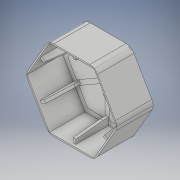
# Autodesk Inventor part: Base v5 - 175
Saved by Autodesk Inventor 2019 (Build 230136000, 136)
## iProperties
Created: 2021-07-14
Part Number: Base v5 - 175
Material: Generic
Document SubType Name: Modeling
Designer: Lix
Density: 1 g/cm^3
Appearance: Default
Author: Lix
## iProperties of the stored document Base v6 - 175_3DPrint.ipt
Created: 2021-08-07
Part Number: Base v6 - 175_3DPrint
Material: Generic
Document SubType Name: Modeling
Designer: Lix
Density: 1 g/cm^3
Appearance: Default
Author: Lix
Autodesk Inventor part; units mm, degrees
sketch "Sketch1" plane through (0, 0, 0) normal (0, 0, 1) x (1, 0, 0)
  line L0 (25.4034, -44) -> (-25.4034, -44)
  line L1 (-25.4034, -44) -> (-50.8068, 0)
  line L2 (-50.8068, 0) -> (-25.4034, 44)
  line L3 (-25.4034, 44) -> (25.4034, 44)
  line L4 (25.4034, 44) -> (50.8068, 0)
  line L5 (50.8068, 0) -> (25.4034, -44)
  point P0 (0, 0)
  point P1 (0, 0)
  point P2 (0, 0)
  dimension "d0" = 88
  constraints: 12 end point, 2 coincident, 1 horizontal, 13 other
  measures "d0" distance between parallel lines of L5 L2
extrude "Extrusion1" add sketch "Sketch1" along normal blind 40
shell "Shell1" thickness 1.5 removed faces 1 at (-8.4678, 14.6667, 40) ; own thickness 1 on faces at (-8.4678, 14.6667, 0)
sketch "Sketch11" plane through (-24.5374, -42.5, 1) normal (0, 0, 1) x (1, 0, 0)
  line L0 (-41.7126, -1) -> (-30.7126, -1)
  line L1 (-30.7126, -1) -> (-30.7126, 86)
  line L2 (-30.7126, 86) -> (-41.7126, 86)
  line L3 (-41.7126, 86) -> (-41.7126, -1)
  line L4 (-41.7126, -1) -> (-30.7126, 86) construction
  line L5 (-30.7126, -1) -> (-41.7126, 86) construction
  line L6 (-1.2126, -1) -> (9.7874, -1)
  line L7 (9.7874, -1) -> (9.7874, 86)
  line L8 (9.7874, 86) -> (-1.2126, 86)
  line L9 (-1.2126, -1) -> (9.7874, 86) construction
  line L10 (9.7874, -1) -> (-1.2126, 86) construction
  line L11 (-1.2126, 86) -> (-1.2126, -1)
  line L12 (39.2874, -1) -> (50.2874, -1)
  line L13 (50.2874, -1) -> (50.2874, 86)
  line L14 (50.2874, 86) -> (39.2874, 86)
  line L15 (39.2874, -1) -> (50.2874, 86) construction
  line L16 (50.2874, -1) -> (39.2874, 86) construction
  line L17 (39.2874, 86) -> (39.2874, -1)
  line L18 (79.7874, -1) -> (90.7874, -1)
  line L19 (90.7874, -1) -> (90.7874, 86)
  line L20 (90.7874, 86) -> (79.7874, 86)
  line L21 (79.7874, -1) -> (90.7874, 86) construction
  line L22 (90.7874, -1) -> (79.7874, 86) construction
  line L23 (79.7874, 86) -> (79.7874, -1)
  line L24 (-36.2126, 42.5) -> (85.2874, 42.5) construction
  line L25 (-18.9626, -28) -> (68.0374, -28)
  line L26 (68.0374, -28) -> (68.0374, -17)
  line L27 (68.0374, -17) -> (-18.9626, -17)
  line L28 (-18.9626, -17) -> (-18.9626, -28)
  line L29 (-18.9626, -28) -> (68.0374, -17) construction
  line L30 (68.0374, -28) -> (-18.9626, -17) construction
  line L31 (24.5374, -22.5) -> (24.5374, 107.5) construction
  line L32 (-18.9626, 102) -> (68.0374, 102)
  line L33 (68.0374, 102) -> (68.0374, 113)
  line L34 (68.0374, 113) -> (-18.9626, 113)
  line L35 (-18.9626, 113) -> (-18.9626, 102)
  line L36 (-18.9626, 102) -> (68.0374, 113) construction
  line L37 (68.0374, 102) -> (-18.9626, 113) construction
  line L38 (-19.9626, 114) -> (69.0374, 114)
  line L39 (69.0374, 114) -> (69.0374, 101)
  line L40 (69.0374, 101) -> (-19.9626, 101)
  line L41 (-19.9626, 101) -> (-19.9626, 114)
  line L42 (-42.7126, 87) -> (-29.7126, 87)
  line L43 (-29.7126, 87) -> (-29.7126, -2)
  line L44 (-29.7126, -2) -> (-42.7126, -2)
  line L45 (-42.7126, -2) -> (-42.7126, 87)
  line L46 (-2.2126, 87) -> (10.7874, 87)
  line L47 (10.7874, 87) -> (10.7874, -2)
  line L48 (10.7874, -2) -> (-2.2126, -2)
  line L49 (-2.2126, -2) -> (-2.2126, 87)
  line L50 (38.2874, 87) -> (51.2874, 87)
  line L51 (51.2874, 87) -> (51.2874, -2)
  line L52 (51.2874, -2) -> (38.2874, -2)
  line L53 (38.2874, -2) -> (38.2874, 87)
  line L54 (78.7874, 87) -> (91.7874, 87)
  line L55 (91.7874, 87) -> (91.7874, -2)
  line L56 (91.7874, -2) -> (78.7874, -2)
  line L57 (78.7874, -2) -> (78.7874, 87)
  line L58 (69.0374, -29) -> (-19.9626, -29)
  line L59 (-19.9626, -29) -> (-19.9626, -16)
  line L60 (-19.9626, -16) -> (69.0374, -16)
  line L61 (69.0374, -16) -> (69.0374, -29)
  line L62 (90.7874, 87) -> (79.7874, 87)
  line L63 (79.7874, 87) -> (79.7874, -2)
  line L64 (79.7874, -2) -> (90.7874, -2)
  line L65 (90.7874, -2) -> (90.7874, 87)
  line L66 (50.2874, 87) -> (39.2874, 87)
  line L67 (39.2874, 87) -> (39.2874, -2)
  line L68 (39.2874, -2) -> (50.2874, -2)
  line L69 (50.2874, -2) -> (50.2874, 87)
  line L70 (69.0374, 113) -> (-19.9626, 113)
  line L71 (-19.9626, 113) -> (-19.9626, 102)
  line L72 (-19.9626, 102) -> (69.0374, 102)
  line L73 (69.0374, 102) -> (69.0374, 113)
  line L74 (-30.7126, 87) -> (-41.7126, 87)
  line L75 (-41.7126, 87) -> (-41.7126, -2)
  line L76 (-41.7126, -2) -> (-30.7126, -2)
  line L77 (-30.7126, -2) -> (-30.7126, 87)
  line L78 (9.7874, 87) -> (-1.2126, 87)
  line L79 (-1.2126, 87) -> (-1.2126, -2)
  line L80 (-1.2126, -2) -> (9.7874, -2)
  line L81 (9.7874, -2) -> (9.7874, 87)
  line L82 (69.0374, -17) -> (-19.9626, -17)
  line L83 (-19.9626, -17) -> (-19.9626, -28)
  line L84 (-19.9626, -28) -> (69.0374, -28)
  line L85 (69.0374, -28) -> (69.0374, -17)
  point P0 (24.5374, 42.5)
  point P1 (4.2874, 42.5)
  point P2 (44.7874, 42.5)
  point P3 (24.5374, 42.5)
  dimension "d138" = 11
  dimension "d139" = 87
  dimension "d142" = 40.5
  dimension "d147" = 130
  dimension "d151" = 1
  dimension "d152" = 1
  dimension "d153" = 1
  dimension "d154" = 1
  dimension "d155" = 1
  dimension "d156" = 1
  constraints: 172 end point, 24 parallel, 14 midpoint, 13 point on line, 12 perpendicular, 11 horizontal, 4 equal length, 1 coincident, 1 collinear, 1 horizontal alignment, 1 vertical, 50 other
  measures "d138" distance of L1.end L2.end
  measures "d139" distance of L2.end L0.start
  measures "d142" distance of L0.end L6.end
  measures "d147" distance of L31.start L31.end
  measures "d151" distance between parallel lines of L34 L38
  measures "d152" distance between parallel lines of L2 L42
  measures "d153" distance between parallel lines of L8 L46
  measures "d154" distance between parallel lines of L14 L50
  measures "d155" distance between parallel lines of L20 L54
  measures "d156" distance between parallel lines of L25 L58
extrude "Extrusion9" [suppressed]
ref_plane "Work Plane1" through (-12.7017, 22, 40) normal (0.8660254, 0.5, 0) x (0, 0, -1)
ref_plane "Work Plane2" through (-25.4034, 0, 0) normal (0, 1, 0) x (1, 0, 0)
ref_plane "Work Plane3" through (-12.7017, -22, 0) normal (-0.8660254, 0.5, 0) x (0, 0, 1)
sketch "Sketch12" plane through (-24.5374, -42.5, 1) normal (0, 0, 1) x (1, 0, 0)
  line L0 (49.0748, 0) -> (0, 0) projected
  line L1 (73.6122, 42.5) -> (49.0748, 0) projected
  line L2 (49.0748, 85) -> (73.6122, 42.5) projected
  line L3 (0, 85) -> (49.0748, 85) projected
  line L4 (-24.5374, 42.5) -> (0, 85) projected
  line L5 (0, 0) -> (-24.5374, 42.5) projected
  point P0 (24.5374, 42.5)
sketch "Sketch4" plane through (-24.5374, -42.5, 1) normal (0, 0, 1) x (1, 0, 0)
  line L0 (49.0748, 0) -> (0, 0) projected
  line L1 (73.6122, 42.5) -> (49.0748, 0) projected
  line L2 (49.0748, 85) -> (73.6122, 42.5) projected
  line L3 (0, 85) -> (49.0748, 85) projected
  line L4 (-24.5374, 42.5) -> (0, 85) projected
  line L5 (0, 0) -> (-24.5374, 42.5) projected
  line L6 (-6.7257, 63.3507) -> (2.8868, 80)
  line L7 (2.8868, 80) -> (22.1117, 80)
  line L8 (49.0748, 85) -> (0, 0) construction
  arc A0 (22.1117, 52.2014) -> (17.3486, 49.4514) centre (24.5374, 42.5) ccw
  line L9 (-6.7257, 63.3507) -> (17.3486, 49.4514)
  line L10 (22.1117, 80) -> (22.1117, 52.2014)
  circle A1 centre (49.6521, 86) radius 2.5
  arc A2 (14.9229, 45.25) -> (14.9229, 39.75) centre (24.5374, 42.5) ccw
  line L11 (-9.1514, 59.1493) -> (14.9229, 45.25)
  line L12 (-9.1514, 25.8507) -> (14.9229, 39.75)
  line L13 (-9.1514, 25.8507) -> (-18.7639, 42.5)
  line L14 (-18.7639, 42.5) -> (-9.1514, 59.1493)
  arc A3 (17.3486, 35.5486) -> (22.1117, 32.7986) centre (24.5374, 42.5) ccw
  line L15 (-6.7257, 21.6493) -> (17.3486, 35.5486)
  line L16 (22.1117, 5) -> (22.1117, 32.7986)
  line L17 (22.1117, 5) -> (2.8868, 5)
  line L18 (2.8868, 5) -> (-6.7257, 21.6493)
  arc A4 (26.963, 32.7986) -> (31.7262, 35.5486) centre (24.5374, 42.5) ccw
  line L19 (26.963, 5) -> (26.963, 32.7986)
  line L20 (55.8005, 21.6493) -> (31.7262, 35.5486)
  line L21 (55.8005, 21.6493) -> (46.188, 5)
  line L22 (46.188, 5) -> (26.963, 5)
  arc A5 (34.1518, 39.75) -> (34.1518, 45.25) centre (24.5374, 42.5) ccw
  line L23 (58.2262, 25.8507) -> (34.1518, 39.75)
  line L24 (58.2262, 59.1493) -> (34.1518, 45.25)
  line L25 (58.2262, 59.1493) -> (67.8387, 42.5)
  line L26 (67.8387, 42.5) -> (58.2262, 25.8507)
  arc A6 (31.7262, 49.4514) -> (26.963, 52.2014) centre (24.5374, 42.5) ccw
  line L27 (55.8005, 63.3507) -> (31.7262, 49.4514)
  line L28 (26.963, 80) -> (26.963, 52.2014)
  line L29 (26.963, 80) -> (46.188, 80)
  line L30 (46.188, 80) -> (55.8005, 63.3507)
  point P0 (-24.5374, 42.5)
  point P1 (0, 0)
  point P2 (49.0748, 0)
  point P3 (73.6122, 42.5)
  point P4 (49.0748, 85)
  dimension "d37" = 5
  dimension "d44" = 10
  dimension "d45" = 60
  dimension "d46" = 90
  dimension "d47" = 90
  dimension "d52" = 5.5
  dimension "d55" = 5
  dimension "d72" = 360
  constraints: 50 end point, 12 point on circle, 7 centre point, 2 equal length, 1 coincident, 1 midpoint, 73 other
  measures "d37" distance between parallel lines of L3 L7
  measures "d44" radius of A0
  measures "d45" angle of L10 L9
  measures "d46" angle of L9 L6
  measures "d47" angle of L10 L7
  measures "d52" distance of L10.end L9.end
  measures "d55" diameter of A1
extrude "Extrusion5" cut sketch "Sketch4" against normal blind 0.01 contours A1 L3 L2 | L2 L3 A1 | L6 L7 L10 A0 L9 | A2 L12 L13 L14 L11 | A3 L16 L17 L18 L15 | A4 L20 L21 L22 L19 | A5 L24 L25 L26 L23 | A6 L28 L29 L30 L27
sketch "Sketch8" plane through (-24.5374, -42.5, 1) normal (0, 0, 1) x (1, 0, 0)
  line L0 (49.0748, 0) -> (0, 0) projected
  line L1 (73.6122, 42.5) -> (49.0748, 0) projected
  line L2 (-24.5374, 42.5) -> (0, 85) projected
  line L3 (0, 0) -> (-24.5374, 42.5) projected
  line L4 (23.0374, 77) -> (26.0374, 77)
  line L5 (26.0374, 77) -> (26.0374, 85)
  line L6 (26.0374, 85) -> (23.0374, 85)
  line L7 (23.0374, 85) -> (23.0374, 77)
  line L8 (0, 85) -> (49.0748, 85) projected
  line L9 (24.5374, 86) -> (24.5374, 85)
  line L10 (58.2262, 25.8507) -> (34.1518, 39.75) projected
  arc A0 (34.1518, 39.75) -> (34.1518, 45.25) centre (24.5374, 42.5) ccw projected
  line L11 (34.1518, 45.25) -> (58.2262, 59.1493) projected
  line L12 (55.8005, 63.3507) -> (31.7262, 49.4514) projected
  arc A1 (31.7262, 49.4514) -> (26.963, 52.2014) centre (24.5374, 42.5) ccw projected
  line L13 (26.963, 52.2014) -> (26.963, 80) projected
  line L14 (26.963, 80) -> (46.188, 80) projected
  line L15 (2.8868, 80) -> (22.1117, 80) projected
  line L16 (22.1117, 80) -> (22.1117, 52.2014) projected
  arc A2 (22.1117, 52.2014) -> (17.3486, 49.4514) centre (24.5374, 42.5) ccw projected
  line L17 (17.3486, 49.4514) -> (-6.7257, 63.3507) projected
  line L18 (-9.1514, 59.1493) -> (14.9229, 45.25) projected
  arc A3 (14.9229, 45.25) -> (14.9229, 39.75) centre (24.5374, 42.5) ccw projected
  line L19 (14.9229, 39.75) -> (-9.1514, 25.8507) projected
  line L20 (-6.7257, 21.6493) -> (17.3486, 35.5486) projected
  arc A4 (17.3486, 35.5486) -> (22.1117, 32.7986) centre (24.5374, 42.5) ccw projected
  line L21 (22.1117, 32.7986) -> (22.1117, 5) projected
  line L22 (22.1117, 5) -> (2.8868, 5) projected
  line L23 (46.188, 5) -> (26.963, 5) projected
  line L24 (26.963, 5) -> (26.963, 32.7986) projected
  arc A5 (26.963, 32.7986) -> (31.7262, 35.5486) centre (24.5374, 42.5) ccw projected
  line L25 (31.7262, 35.5486) -> (55.8005, 21.6493) projected
  arc A6 (47.3608, 85) -> (49.9317, 83.5157) centre (49.6521, 86) ccw projected
  line L26 (0, 85) -> (47.3608, 85) projected
  line L27 (46.188, 80) -> (55.8005, 63.3507) projected
  line L28 (49.9317, 83.5157) -> (73.6122, 42.5) projected
  line L29 (55.8005, 21.6493) -> (46.188, 5) projected
  line L30 (58.2262, 59.1493) -> (67.8387, 42.5) projected
  line L31 (67.8387, 42.5) -> (58.2262, 25.8507) projected
  line L32 (2.8868, 5) -> (-6.7257, 21.6493) projected
  line L33 (-6.7257, 63.3507) -> (2.8868, 80) projected
  line L34 (-9.1514, 25.8507) -> (-18.7639, 42.5) projected
  line L35 (-18.7639, 42.5) -> (-9.1514, 59.1493) projected
  point P0 (24.5374, 42.5)
  dimension "d57" = 3
  dimension "d58" = 8
  constraints: 10 end point, 2 midpoint, 2 parallel, 1 coincident, 1 horizontal, 1 perpendicular, 1 vertical
  measures "d57" distance of L4.start L4.end
  measures "d58" distance of L4.end L5.end
extrude "Extrusion6" add sketch "Sketch8" along normal blind 36 contours L6 L5 L4 L7
sketch "Sketch9" plane through (1.5, 34.5, 1) normal (1, 0, 0) x (0, 0, -1)
  line L0 (0, 0) -> (0, 8) projected
  line L1 (0, 0) -> (-36, 0) projected
  line L2 (-36, 8) -> (-36, 0) projected
  line L3 (0, 8) -> (-36, 8) projected
  line L4 (-36, 8) -> (-36, 0) projected
  line L5 (-36, 0) -> (-6, 0)
  line L6 (0, 0) -> (-36, 0) projected
  line L7 (-6, 0) -> (-36, 3)
  line L8 (-36, 3) -> (-36, 0)
  point P0 (1, -34.5)
  point P1 (-36, 8)
  dimension "d77" = 3
  dimension "d78" = 30
  constraints: 6 end point, 3 point on line, 1 collinear, 1 perpendicular
  measures "d77" distance of L7.end L5.start
  measures "d78" distance of L5.start L5.end
extrude "Extrusion8" cut sketch "Sketch9" against normal blind 20 contours L1 L2 L7
pattern_circular "Circular Pattern1" count 6 over 360 about axis through (0, 0, 1) along (0, 0, -1) of "Extrusion6", "Extrusion8"
fillet "Fillet1" [suppressed]
fillet "Fillet2" radius 10 7 edges at (50.8068, 0, 20) (25.4034, 44, 0.495) (25.4034, 44, 20.5) (-25.4034, 44, 20) (25.4034, -44, 20) (-50.8068, 0, 20) (-25.4034, -44, 20)
fillet "Fillet4" radius 2 5 edges at (-7.1888, 6.9514, 0.995) (-2.4257, 9.7014, 0.995) (-2.4257, 37.5, 0.995) (-21.6506, 37.5, 0.995) (-31.2631, 20.8507, 0.995)
sketch "Sketch5" plane through (-19.6299, 44, 0) normal (0, 1, 0) x (1, 0, 0)
  line L0 (0, 0) -> (39.2598, 0) projected
  line L1 (0, -40) -> (0, 0) projected
  point P0 (19.6299, 0)
  point P1 (19.6299, -20)
  point P2 (19.6299, 0)
  point P3 (0, -20)
  constraints: 2 midpoint, 1 horizontal alignment, 1 vertical alignment
sketch "Sketch6" plane through (28.2902, 39, 40) normal (0.8660254, 0.5, 0) x (0, 0, -1)
  line L0 (40, 8.6603) -> (0, 8.6603) projected
  point P0 (40, -19.6299)
  point P1 (20, -19.6299)
  point P2 (20, 8.6603)
  constraints: 1 horizontal alignment, 1 midpoint, 1 vertical alignment
sketch "Sketch7" plane through (28.2902, -39, 40) normal (0.8660254, -0.5, 0) x (0, 0, -1)
  line L0 (0, -8.6603) -> (40, -8.6603) projected
  point P0 (40, 19.6299)
  point P1 (20, 19.6299)
  point P2 (20, -8.6603)
  constraints: 1 horizontal alignment, 1 midpoint, 1 vertical alignment
sketch "Sketch13" plane through (0, 0, 40) normal (0, 0, 1) x (1, 0, 0)
  line L0 (-66.25, -43.5) -> (-55.25, -43.5) projected
  line L1 (-55.25, -43.5) -> (-55.25, 43.5) projected
  line L2 (-55.25, 43.5) -> (-66.25, 43.5) projected
  line L3 (-66.25, 43.5) -> (-66.25, -43.5) projected
  line L4 (-25.75, -43.5) -> (-14.75, -43.5) projected
  line L5 (-14.75, -43.5) -> (-14.75, 43.5) projected
  line L6 (-14.75, 43.5) -> (-25.75, 43.5) projected
  line L7 (-25.75, 43.5) -> (-25.75, -43.5) projected
  line L8 (-43.5, 59.5) -> (43.5, 59.5) projected
  line L9 (43.5, 59.5) -> (43.5, 70.5) projected
  line L10 (43.5, 70.5) -> (-43.5, 70.5) projected
  line L11 (-43.5, 70.5) -> (-43.5, 59.5) projected
  line L12 (14.75, -43.5) -> (25.75, -43.5) projected
  line L13 (25.75, -43.5) -> (25.75, 43.5) projected
  line L14 (25.75, 43.5) -> (14.75, 43.5) projected
  line L15 (14.75, 43.5) -> (14.75, -43.5) projected
  line L16 (55.25, -43.5) -> (66.25, -43.5) projected
  line L17 (66.25, -43.5) -> (66.25, 43.5) projected
  line L18 (66.25, 43.5) -> (55.25, 43.5) projected
  line L19 (55.25, 43.5) -> (55.25, -43.5) projected
  line L20 (-43.5, -70.5) -> (43.5, -70.5) projected
  line L21 (43.5, -70.5) -> (43.5, -59.5) projected
  line L22 (43.5, -59.5) -> (-43.5, -59.5) projected
  line L23 (-43.5, -59.5) -> (-43.5, -70.5) projected
  arc A0 (-28.2902, -39) -> (-19.6299, -44) centre (-19.6299, -34) ccw projected
  line L24 (-19.6299, -44) -> (19.6299, -44) projected
  arc A1 (19.6299, -44) -> (28.2902, -39) centre (19.6299, -34) ccw projected
  line L25 (28.2902, -39) -> (47.9201, -5) projected
  arc A2 (47.9201, -5) -> (47.9201, 5) centre (39.2598, 0) ccw projected
  line L26 (47.9201, 5) -> (28.2902, 39) projected
  arc A3 (28.2902, 39) -> (19.6299, 44) centre (19.6299, 34) ccw projected
  line L27 (19.6299, 44) -> (-19.6299, 44) projected
  arc A4 (-19.6299, 44) -> (-28.2902, 39) centre (-19.6299, 34) ccw projected
  line L28 (-28.2902, 39) -> (-47.9201, 5) projected
  arc A5 (-47.9201, 5) -> (-47.9201, -5) centre (-39.2598, 0) ccw projected
  line L29 (-47.9201, -5) -> (-28.2902, -39) projected
  line L30 (-24.5374, -42.5) -> (-49.0748, 0) projected
  line L31 (-49.0748, 0) -> (-24.5374, 42.5) projected
  line L32 (-24.5374, 42.5) -> (24.5374, 42.5) projected
  line L33 (24.5374, 42.5) -> (49.0748, 0) projected
  line L34 (49.0748, 0) -> (24.5374, -42.5) projected
  line L35 (24.5374, -42.5) -> (-24.5374, -42.5) projected
  line L36 (1.5, -37.5) -> (-1.5, -37.5) projected
  line L37 (-1.5, -37.5) -> (-1.5, -42.5) projected
  line L38 (1.5, -42.5) -> (-1.5, -42.5) projected
  line L39 (1.5, -42.5) -> (1.5, -37.5) projected
  line L40 (-31.726, -20.049) -> (-33.226, -17.451) projected
  line L41 (-33.226, -17.451) -> (-37.5561, -19.951) projected
  line L42 (-36.0561, -22.549) -> (-37.5561, -19.951) projected
  line L43 (-36.0561, -22.549) -> (-31.726, -20.049) projected
  line L44 (-29.1279, -18.549) -> (-31.726, -20.049) projected
  line L45 (-30.6279, -15.951) -> (-29.1279, -18.549) projected
  line L46 (-33.226, -17.451) -> (-30.6279, -15.951) projected
  line L47 (-31.726, -20.049) -> (-33.226, -17.451) projected
  line L48 (1.5, -34.5) -> (1.5, -37.5) projected
  line L49 (-1.5, -34.5) -> (1.5, -34.5) projected
  line L50 (-1.5, -37.5) -> (-1.5, -34.5) projected
  line L51 (1.5, -37.5) -> (-1.5, -37.5) projected
  line L52 (-33.226, 17.451) -> (-31.726, 20.049) projected
  line L53 (-31.726, 20.049) -> (-36.0561, 22.549) projected
  line L54 (-37.5561, 19.951) -> (-36.0561, 22.549) projected
  line L55 (-37.5561, 19.951) -> (-33.226, 17.451) projected
  line L56 (-30.6279, 15.951) -> (-33.226, 17.451) projected
  line L57 (-29.1279, 18.549) -> (-30.6279, 15.951) projected
  line L58 (-31.726, 20.049) -> (-29.1279, 18.549) projected
  line L59 (-33.226, 17.451) -> (-31.726, 20.049) projected
  line L60 (-1.5, 37.5) -> (1.5, 37.5) projected
  line L61 (1.5, 37.5) -> (1.5, 42.5) projected
  line L62 (-1.5, 42.5) -> (1.5, 42.5) projected
  line L63 (-1.5, 42.5) -> (-1.5, 37.5) projected
  line L64 (-1.5, 34.5) -> (-1.5, 37.5) projected
  line L65 (1.5, 34.5) -> (-1.5, 34.5) projected
  line L66 (1.5, 37.5) -> (1.5, 34.5) projected
  line L67 (-1.5, 37.5) -> (1.5, 37.5) projected
  line L68 (31.726, 20.049) -> (33.226, 17.451) projected
  line L69 (33.226, 17.451) -> (37.5561, 19.951) projected
  line L70 (36.0561, 22.549) -> (37.5561, 19.951) projected
  line L71 (36.0561, 22.549) -> (31.726, 20.049) projected
  line L72 (29.1279, 18.549) -> (31.726, 20.049) projected
  line L73 (30.6279, 15.951) -> (29.1279, 18.549) projected
  line L74 (33.226, 17.451) -> (30.6279, 15.951) projected
  line L75 (31.726, 20.049) -> (33.226, 17.451) projected
  line L76 (33.226, -17.451) -> (31.726, -20.049) projected
  line L77 (31.726, -20.049) -> (36.0561, -22.549) projected
  line L78 (37.5561, -19.951) -> (36.0561, -22.549) projected
  line L79 (37.5561, -19.951) -> (33.226, -17.451) projected
  line L80 (30.6279, -15.951) -> (33.226, -17.451) projected
  line L81 (29.1279, -18.549) -> (30.6279, -15.951) projected
  line L82 (31.726, -20.049) -> (29.1279, -18.549) projected
  line L83 (33.226, -17.451) -> (31.726, -20.049) projected
  point P0 (0, 0)
body "Solid1"
